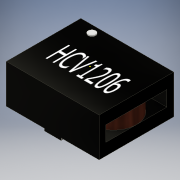
# Autodesk Inventor part: HCV1206
Saved by Autodesk Inventor 2019.4 (Build 234330000, 330)
## iProperties
Created: 2019-12-30
Part Number: HCV1206
Material: Generic
Document SubType Name: Modeling
Designer: Jorian Bruslind
Density: 1 g/cm^3
Appearance: Gunmetal
Author: Jorian Bruslind
Autodesk Inventor part; units mm, degrees
ref_plane "YZ Plane" through (0, 0, 0) normal (1, 0, 0) x (0, 1, 0)
ref_plane "XZ Plane" through (0, 0, 0) normal (0, 1, 0) x (-1, 0, 0)
ref_plane "XY Plane" through (0, 0, 0) normal (0, 0, 1) x (1, 0, 0)
sketch "Sketch1" plane through (0, 0, 0) normal (0, 1, 0) x (-1, 0, 0)
  line L0 (-6.1, 4.9) -> (6.1, 4.9)
  line L1 (6.1, 4.9) -> (6.1, -4.9)
  line L2 (6.1, -4.9) -> (-6.1, -4.9)
  line L3 (-6.1, -4.9) -> (-6.1, 4.9)
  line L4 (-6.1, 4.9) -> (6.1, -4.9) construction
  line L5 (6.1, 4.9) -> (-6.1, -4.9) construction
  point P0 (0, 0)
  dimension "d0" = 12.2
  dimension "d1" = 9.8
  constraints: 12 end point, 2 midpoint, 2 parallel, 1 horizontal, 1 perpendicular
  measures "d0" distance of L1.end L2.end
  measures "d1" distance of L0.end L1.end
extrude "Extrusion1" add sketch "Sketch1" along normal blind 5.1
sketch "Sketch2" plane through (6.1, 0, 4.9) normal (1, 0, 0) x (0, 0, -1)
  line L0 (4.9, 0) -> (4.9, 2.55)
  line L1 (0, 0) -> (0, 5.1) projected
  line L2 (8.9, 1.55) -> (0.9, 1.55)
  line L3 (0.9, 1.55) -> (0.9, 3.55)
  line L4 (0.9, 3.55) -> (8.9, 3.55)
  line L5 (8.9, 3.55) -> (8.9, 1.55)
  line L6 (8.9, 1.55) -> (0.9, 3.55) construction
  line L7 (0.9, 1.55) -> (8.9, 3.55) construction
  dimension "d4" = 2.55
  dimension "d5" = 8
  dimension "d6" = 2
  constraints: 14 end point, 3 parallel, 2 midpoint, 1 horizontal, 1 perpendicular
  measures "d4" distance of L0.start L0.end
  measures "d5" distance of L3.end L4.end
  measures "d6" distance of L2.end L3.end
extrude "Extrusion2" cut sketch "Sketch2" against normal up to next
sketch "Sketch3" plane through (6.1, 1.55, 4) normal (0, 1, 0) x (1, 0, 0)
  line L0 (-12.2, 8.9) -> (-12.2, -0.9) projected
  line L1 (-12.2, 4) -> (-9.2, 4)
  line L2 (0, 0) -> (0, 8) projected
  line L3 (0, 4) -> (-3, 4)
  circle A0 centre (-3, 4) radius 3
  circle A1 centre (-9.2, 4) radius 3
  point P0 (-6.1, 4)
  dimension "d9" = 3
  dimension "d10" = 3
  dimension "d11" = 6
  dimension "d12" = 6
  constraints: 4 end point, 2 centre point, 2 coincident, 2 horizontal, 2 midpoint
  measures "d9" distance of L1.start L1.end
  measures "d10" distance of L3.start L3.end
  measures "d11" diameter of A0
  measures "d12" diameter of A1
extrude "Extrusion3" add sketch "Sketch3" along normal up to next
sketch "Sketch4" plane through (0, 0, 0) normal (0, -1, 0) x (1, 0, 0)
  line L0 (6.1, 4.9) -> (-6.1, 4.9) projected
  line L1 (0, 4.9) -> (0, 4.25)
  line L2 (1.1, 3.6) -> (-1.1, 3.6)
  line L3 (-1.1, 3.6) -> (-1.1, 4.9)
  line L4 (-1.1, 4.9) -> (1.1, 4.9)
  line L5 (1.1, 4.9) -> (1.1, 3.6)
  line L6 (1.1, 3.6) -> (-1.1, 4.9) construction
  line L7 (-1.1, 3.6) -> (1.1, 4.9) construction
  line L8 (6.1, -4.9) -> (-6.1, -4.9) projected
  line L9 (-6.1, -4.9) -> (-4.75, -4.9)
  line L10 (-4.75, -4.9) -> (-3.65, -4.9)
  line L11 (-3.65, -4.9) -> (-3.65, -3.9)
  line L12 (-3.65, -4.9) -> (-2.65, -4.9) construction
  line L13 (-2.55, -2.9) -> (-4.75, -2.9)
  line L14 (-4.75, -2.9) -> (-4.75, -4.9)
  line L15 (-4.75, -4.9) -> (-2.55, -4.9)
  line L16 (-2.55, -4.9) -> (-2.55, -2.9)
  line L17 (-2.55, -2.9) -> (-4.75, -4.9) construction
  line L18 (-4.75, -2.9) -> (-2.55, -4.9) construction
  line L19 (4.75, -2.9) -> (2.55, -2.9)
  line L20 (4.75, -4.9) -> (4.75, -2.9)
  line L21 (3.65, -4.9) -> (4.65, -4.9) construction
  line L22 (2.55, -2.9) -> (2.55, -4.9)
  line L23 (2.55, -4.9) -> (4.75, -4.9)
  point P0 (0, 0)
  dimension "d15" = 0.65
  dimension "d16" = 2.2
  dimension "d17" = 1.3
  dimension "d18" = 1.35
  dimension "d19" = 1.1
  dimension "d20" = 1
  dimension "d21" = 90
  dimension "d22" = 2.2
  dimension "d23" = 2
  dimension "d26" = 7.3
  constraints: 44 end point, 5 midpoint, 4 horizontal, 4 parallel, 3 perpendicular, 2 point on line, 2 vertical, 11 other
  measures "d15" distance of L1.start L1.end
  measures "d16" distance of L3.end L4.end
  measures "d17" distance of L2.end L3.end
  measures "d18" distance of L8.end L9.end
  measures "d19" distance of L9.end L10.end
  measures "d20" distance of L10.end L11.end
  measures "d21" angle of L12 L11
  measures "d22" distance of L15.end L9.end
  measures "d23" distance of L9.end L13.end
  measures "d26" distance of L13.start L19.start
extrude "Extrusion4" add sketch "Sketch4" along normal blind 0.3
sketch "Sketch5" plane through (0, 5.1, 0) normal (0, 1, 0) x (1, 0, 0)
  line L0 (6.1, 4.9) -> (-6.1, 4.9) projected
  line L1 (-6.1, 4.9) -> (-3.65, 4.9)
  line L2 (-3.65, 4.9) -> (-3.65, 3.9)
  circle A0 centre (-3.65, 3.9) radius 0.5
  point P0 (0, 0)
  dimension "d33" = 2.45
  dimension "d34" = 1
  dimension "d35" = 1
  constraints: 4 end point, 1 centre point, 1 coincident, 1 perpendicular, 1 point on line
  measures "d33" distance of L0.end L1.end
  measures "d34" distance of L1.end L2.end
  measures "d35" diameter of A0
extrude "Extrusion5" add sketch "Sketch5" along normal blind 0.1
sketch "Sketch6" plane through (0, 5.1, 0) normal (0, 1, 0) x (1, 0, 0)
  line L0 (-4.0529, 1.1605) -> (0.3424, 1.1605) construction
  line L1 (0.3424, 1.1605) -> (0.3424, 0.2782) construction
  line L2 (0.3424, 0.2782) -> (-4.0529, 0.2782) construction
  line L3 (-4.0529, 0.2782) -> (-4.0529, 1.1605) construction
  point P0 (0, 0)
  dimension "d1" = 9.8
  constraints: 2 other
body "Solid1"
